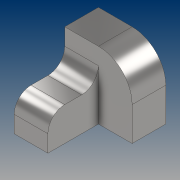
# Autodesk Inventor part: 45
Saved by Autodesk Inventor 2020.2 (Build 242310000, 310)
## iProperties
Created: 2020-09-17
Part Number: 45
Material: 鋼、碳鋼
Document SubType Name: Modeling
Designer: user
Density: 7.85 g/cm^3
Appearance: 半拋光
Mass: 331.923 g
Surface Area: 82.8496 cm^2
Volume: 42.2832 cm^3
Author: user
Autodesk Inventor part; units mm, degrees
ref_plane "YZ Plane" through (0, 0, 0) normal (1, 0, 0) x (0, 1, 0)
ref_plane "XZ Plane" through (0, 0, 0) normal (0, 1, 0) x (-1, 0, 0)
ref_plane "XY Plane" through (0, 0, 0) normal (0, 0, 1) x (1, 0, 0)
sketch "草圖1" plane through (0, 0, 0) normal (0, 1, 0) x (-1, 0, 0)
  line L0 (0, 0) -> (-20, 0)
  line L1 (-20, 0) -> (-20, 50)
  line L2 (-20, 50) -> (0, 50)
  line L3 (0, 50) -> (0, 0)
  line L4 (0, 0) -> (-40, 0)
  line L5 (-40, 0) -> (-40, 20)
  line L6 (-40, 20) -> (0, 20)
  line L7 (0, 20) -> (0, 0)
  point P0 (0, 20)
  dimension "d0" = 20
  dimension "d1" = 20
  dimension "d2" = 50
  dimension "d3" = 40
  constraints: 16 end point, 4 parallel, 2 horizontal, 2 perpendicular
  measures "d0" distance of L1.end L2.end
  measures "d1" distance of L4.end L5.end
  measures "d2" distance of L2.end L0.start
  measures "d3" distance of L0.start L4.end
extrude "擠出1" add sketch "草圖1" along normal blind 20 contours L0 L1 L6 L3 | L6 L1 L2 L3
extrude "擠出2" add sketch "草圖1" along normal blind 40 contours L0 L1 L6 L3 | L4 L5 L6 L1
fillet "圓角1" radius 20 1 edges at (40, 40, 10)
fillet "圓角2" radius 10 2 edges at (10, 20, 50) (10, 20, 20)
